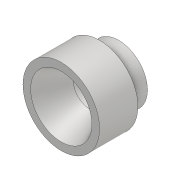
# Autodesk Inventor part: nut
Saved by Autodesk Inventor 2018.1 (Build 221171000, 171)
## iProperties
Created: 2019-06-27
Part Number: nut
Material: Сталь, литейная
Document SubType Name: Modeling
Designer: Boss
Mass: 1.31768 g
Surface Area: 2.78878 cm^2
Volume: 0.167858 cm^3
Density: 7.85 g/cm^3
Appearance: С умеренной полировкой
Author: Boss
Autodesk Inventor part; units mm, degrees
ref_plane "YZ Plane" through (0, 0, 0) normal (1, 0, 0) x (0, 1, 0)
ref_plane "XZ Plane" through (0, 0, 0) normal (0, 1, 0) x (-1, 0, 0)
ref_plane "XY Plane" through (0, 0, 0) normal (0, 0, 1) x (1, 0, 0)
sketch "Эскиз1" plane through (0, 0, 0) normal (0, 0, 1) x (1, 0, 0)
  line L0 (69.1759, 4.9444) -> (70.4259, 4.9444)
  line L1 (70.4259, 4.9444) -> (70.4259, 2.9444)
  line L2 (67.4259, 4.9444) -> (67.4259, 0)
  line L3 (69.1759, 4.9444) -> (69.1759, 1.9444)
  line L4 (70.4259, 2.9444) -> (71.4259, 2.9444)
  line L5 (71.4259, 2.9444) -> (71.4259, -1.0556)
  line L6 (71.4259, -1.0556) -> (70.6259, -1.0556)
  line L7 (70.6259, -1.0556) -> (69.1759, 1.9444)
  point P0 (0, 0)
  dimension "d0" = 6
  dimension "d1" = 8
  dimension "d2" = 2
  dimension "d3" = 4
  dimension "d4" = 3
  dimension "d5" = 0.8
  dimension "d6" = 3.5
  constraints: 16 end point, 3 perpendicular, 1 parallel, 1 point on line, 1 vertical
  measures "d0" diameter of L1 L2
  measures "d1" diameter of L5 L2
  measures "d2" distance of L0.end L1.end
  measures "d3" distance of L4.end L5.end
  measures "d4" distance of L0.start L3.end
  measures "d5" distance of L5.end L6.end
  measures "d6" diameter of L3 L2
revolve "Вращение1" add sketch "Эскиз1" angle 360 about axis through (67.4259, 4.9444, 0) along (0, -1, 0)
chamfer "Фаска1" distance 0.5 angle 45 1 edges at (65.6759, 4.9444, 0)
